Autodesk Fusion 360 part; units mm, degrees
(part 4 of 4)
equation "d102 = d103"
equation "d104 = d103"
equation "d105 = d103"
equation "d106 = d103"
equation "d107 = d103"
equation "d108 = d103"
equation "d118 = ( d114 - d117 ) / 2"
equation "d119 = ( d113 - d116 ) / 2 + 0.25 mm"
equation "d146 = 13 mm - 2 * 0.845 mm"
equation "d150 = 2 mm + 2.25 mm"
equation "d166 = 4 mm - 0.55 mm"
equation "d202 = d203"
equation "d232 = d230"
equation "d233 = d232"
equation "d246 = 19.95 mm - 0.5 mm"
equation "d248 = d243"
equation "d249 = d247"
equation "d250 = d242"
named bodies: "Right frame", "Left frame"
